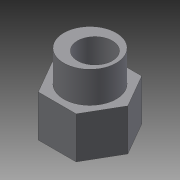
# Autodesk Inventor part: Eccentric_Spacer
Saved by Autodesk Inventor 2014 (Build 180170000, 170)
## iProperties
Created: 2014-08-25
Part Number: Eccentric_Spacer
Material: Generic
Document SubType Name: Modeling
Designer: ThatOtherGuy
Density: 1 g/cm^3
Appearance: Default
Author: ThatOtherGuy
Autodesk Inventor part; units mm, degrees
ref_plane "YZ Plane" through (0, 0, 0) normal (1, 0, 0) x (0, 1, 0)
ref_plane "XZ Plane" through (0, 0, 0) normal (0, 1, 0) x (-1, 0, 0)
ref_plane "XY Plane" through (0, 0, 0) normal (0, 0, 1) x (1, 0, 0)
sketch "Sketch1" plane through (0, 0, 0) normal (0, 0, 1) x (1, 0, 0)
  circle A0 centre (0, 0) radius 4
  line L0 (2.8868, 5) -> (5.7735, 0)
  line L1 (5.7735, 0) -> (2.8868, -5)
  line L2 (2.8868, -5) -> (-2.8868, -5)
  line L3 (-2.8868, -5) -> (-5.7735, 0)
  line L4 (-5.7735, 0) -> (-2.8868, 5)
  line L5 (-2.8868, 5) -> (2.8868, 5)
  circle A1 centre (0.75, 0) radius 2.65
  dimension "d0" = 8
  dimension "d2" = 10
  dimension "d3" = 5.3
  dimension "d4" = 0.75
  constraints: 12 end point, 2 centre point, 2 coincident, 1 horizontal, 1 horizontal alignment, 13 other
  measures "d0" diameter of A0
  measures "d2" distance between parallel lines of L2 L5
  measures "d3" diameter of A1
  measures "d4" distance of point (0, 0) A1.centre
extrude "Extrusion1" add sketch "Sketch1" along normal blind 6.35 contours A0 | L0 L1 L2 L3 L4 L5
sketch "Sketch2" plane through (0, 0, 6.35) normal (0, 0, 1) x (1, 0, 0)
  circle A0 centre (0.75, 0) radius 2.65 projected
  circle A1 centre (0, 0) radius 4
  line L0 (4.0415, 7) -> (8.0829, 0)
  line L1 (8.0829, 0) -> (4.0415, -7)
  line L2 (4.0415, -7) -> (-4.0415, -7)
  line L3 (-4.0415, -7) -> (-8.0829, 0)
  line L4 (-8.0829, 0) -> (-4.0415, 7)
  line L5 (-4.0415, 7) -> (4.0415, 7)
  circle A2 centre (0.75, 0) radius 2.65
  dimension "d7" = 8
  dimension "d8" = 14
  dimension "d9" = 5.3
  constraints: 12 end point, 4 coincident, 2 centre point, 1 horizontal, 1 horizontal alignment, 13 other
  measures "d7" diameter of A1
  measures "d8" distance between parallel lines of L2 L5
  measures "d9" diameter of A2
extrude "Extrusion2" add sketch "Sketch2" along normal blind 4.7625 contours A1
body "Solid1"
